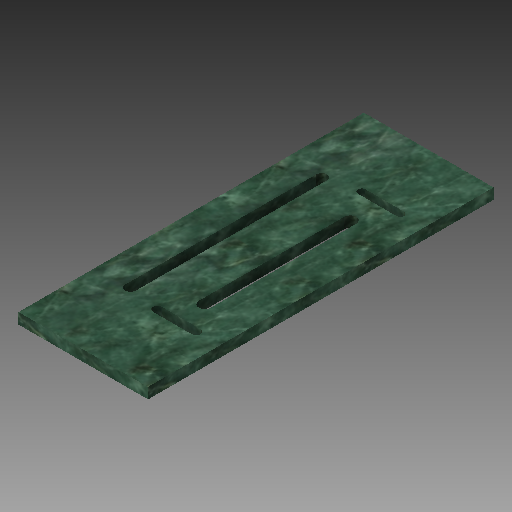
# Autodesk Inventor part: top bottom frame
Saved by Autodesk Inventor 2017 (Build 210142000, 142)
## iProperties
Created: 2019-12-31
Part Number: top bottom frame
Material: LCP Plastic
Document SubType Name: Modeling
Designer: Admin
Density: 1.626 g/cm^3
Appearance: Green Polished
Mass: 17.8976 g
Surface Area: 87.0833 cm^2
Volume: 11.0071 cm^3
Author: Admin
Autodesk Inventor part; units mm, degrees
ref_plane "YZ Plane" through (0, 0, 0) normal (1, 0, 0) x (0, 1, 0)
ref_plane "XZ Plane" through (0, 0, 0) normal (0, 1, 0) x (-1, 0, 0)
ref_plane "XY Plane" through (0, 0, 0) normal (0, 0, 1) x (1, 0, 0)
sketch "Sketch1" plane through (0, 0, 0) normal (0, 1, 0) x (-1, 0, 0)
  line L0 (-12.7, -74.0508) -> (25.4, -74.0508)
  line L1 (25.4, -74.0508) -> (25.4, 27.5492)
  line L2 (25.4, 27.5492) -> (-12.7, 27.5492)
  line L3 (-12.7, 27.5492) -> (-12.7, -74.0508)
  line L4 (-12.7, -74.0508) -> (25.4, 27.5492) construction
  line L5 (25.4, -74.0508) -> (-12.7, 27.5492) construction
  point P0 (0, 0)
  point P1 (6.35, -23.2508)
  dimension "d0" = 38.1
  dimension "d1" = 101.6
  constraints: 12 end point, 2 midpoint, 2 parallel, 1 horizontal, 1 perpendicular
  measures "d0" distance of L1.end L2.end
  measures "d1" distance of L0.end L1.end
extrude "Extrusion1" add sketch "Sketch1" along normal blind 3.175
sketch "Sketch2" plane through (0, 3.175, 0) normal (0, 1, 0) x (1, 0, 0)
  line L0 (0, 1.8272) -> (0, 44.6744) construction
  line L1 (1.7578, 1.8272) -> (1.7578, 44.6744)
  line L2 (-1.7578, 44.6744) -> (-1.7578, 1.8272)
  arc A0 (-1.7578, 1.8272) -> (1.7578, 1.8272) centre (0, 1.8272) ccw
  arc A1 (1.7578, 44.6744) -> (-1.7578, 44.6744) centre (0, 44.6744) ccw
  line L3 (-15.1613, -4.8746) -> (-15.1613, 51.3761) construction
  line L4 (-13.6232, -4.8746) -> (-13.6232, 51.3761)
  line L5 (-16.6994, 51.3761) -> (-16.6994, -4.8746)
  arc A2 (-16.6994, -4.8746) -> (-13.6232, -4.8746) centre (-15.1613, -4.8746) ccw
  arc A3 (-13.6232, 51.3761) -> (-16.6994, 51.3761) centre (-15.1613, 51.3761) ccw
  line L6 (5.713, -6.4127) -> (-5.713, -6.4127) construction
  line L7 (5.713, -5.1314) -> (-5.713, -5.1314)
  line L8 (-5.713, -7.6939) -> (5.713, -7.6939)
  arc A4 (5.713, -7.6939) -> (5.713, -5.1314) centre (5.713, -6.4127) ccw
  arc A5 (-5.713, -5.1314) -> (-5.713, -7.6939) centre (-5.713, -6.4127) ccw
  line L9 (5.713, 53.6139) -> (-5.713, 53.6139) construction
  line L10 (5.713, 54.7126) -> (-5.713, 54.7126)
  line L11 (-5.713, 52.5153) -> (5.713, 52.5153)
  arc A6 (5.713, 52.5153) -> (5.713, 54.7126) centre (5.713, 53.6139) ccw
  arc A7 (-5.713, 54.7126) -> (-5.713, 52.5153) centre (-5.713, 53.6139) ccw
  line L12 (12.7, -27.5492) -> (12.7, 74.0508) projected
  line L13 (-25.4, 74.0508) -> (-25.4, -27.5492) projected
  point P0 (0, 0)
  point P1 (0, 23.2508)
  point P2 (-15.1613, 23.2508)
  point P3 (0, -6.4127)
  point P4 (0, 53.6139)
  point P5 (12.7, 23.2508)
  point P6 (-25.4, 23.2508)
  constraints: 32 end point, 16 point on circle, 16 tangent, 8 centre point, 6 midpoint, 6 parallel, 2 horizontal alignment, 2 vertical alignment, 1 perpendicular, 1 vertical
extrude "Extrusion2" cut sketch "Sketch2" against normal blind 3.175
body "Solid1"
